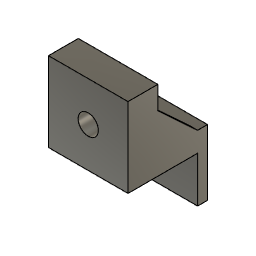
rocker_mount (Autodesk Fusion 360 design; units mm, degrees)
Autodesk Fusion 360 part; units mm, degrees
note: some values were not read from the file. Chosen so that the rebuilt part matches the saved one: a direction.
sketch "Sketch1" plane through (0, 0, 0) normal (1, 0, 0) x (0, 1, 0)
  line L0 (0, 0) -> (35, 0)
  line L1 (35, 0) -> (35, -23)
  line L2 (35, -23) -> (40, -23)
  line L3 (0, 0) -> (0, 10)
  line L4 (15, 30.2) -> (15, 10)
  line L5 (15, 10) -> (40, 10)
  line L6 (40, 10) -> (40, -23)
  line L7 (0, 10) -> (0, 30)
  line L8 (0, 30) -> (0, 40)
  line L9 (0, 40) -> (15, 40)
  line L10 (15, 40) -> (15, 30.2)
  line L11 (15, 10) -> (15, 28.5) construction
  line L12 (15, 28.5) -> (35, 10)
  dimension "d1" = 35
  dimension "d2" = 23
  dimension "d3" = 5
  dimension "d4" = 10
  dimension "d8" = 20.2
  dimension "d9" = 20
  dimension "d10" = 10
  dimension "d19" = 18.5
  constraint coincident L0.start L3.start
  constraint horizontal L0
  constraint perpendicular L0 L1
  constraint perpendicular L1 L2
  constraint perpendicular L0 L3
  constraint perpendicular L0 L4
  constraint perpendicular L4 L5
  constraint perpendicular L2 L6
  constraint parallel L3 L7
  constraint parallel L7 L8
  constraint perpendicular L4 L9
  constraint perpendicular L9 L10
  constraint coincident L4 L11.end
  constraint coincident L5 L12.end
  measures "d1" distance of L0.start L0.end
  measures "d2" distance of L0.end L1.end
  measures "d3" distance of L1.end L2.end
  measures "d4" distance of L0.start L3.end
  measures "d8" distance of L4.start L4.end
  measures "d9" distance of L3.end L7.end
  measures "d10" distance of L7.end L8.end
  measures "d19" distance of L4.end L11.end
extrude "Extrude1" add sketch "Sketch1" along normal blind 40 contours L0 L1 L2 L3 L4 L5 L6 L7 L8 L9 L10
sketch "Sketch2" plane through (0, 0, 0) normal (0, -1, 0) x (1, 0, 0)
  line L0 (0, 40) -> (0, 0)
  line L1 (0, 0) -> (40, 0)
  line L2 (40, 0) -> (40, 40)
  line L3 (40, 40) -> (0, 40)
  line L4 (29.815, 20) -> (24.9075, 28.5)
  line L5 (24.9075, 28.5) -> (15.0925, 28.5)
  line L6 (15.0925, 28.5) -> (10.185, 20)
  line L7 (10.185, 20) -> (15.0925, 11.5)
  line L8 (15.0925, 11.5) -> (24.9075, 11.5)
  line L9 (24.9075, 11.5) -> (29.815, 20)
  line L10 (0, 20) -> (40, 20) construction
  line L11 (20, 40) -> (20, 0) construction
  circle A0 centre (20, 20) radius 5.1
  line L12 (0, 0) -> (0, -11.5) construction
  line L13 (0, -11.5) -> (10, -11.5) construction
  line L14 (10, -11.5) -> (20, -11.5) construction
  circle A1 centre (20, -11.5) radius 2.1
  point P0 (20, 20)
  point P1 (20, 20)
  dimension "d13" = 8.5
  dimension "d14" = 10.2
  dimension "d25" = 11.5
  dimension "d26" = 10
  dimension "d27" = 4.2
  constraint parallel L3 L5
  constraint midpoint L0 L10.start
  constraint midpoint L2 L10.end
  constraint midpoint L3 L11.start
  constraint midpoint L1 L11.end
  constraint midpoint L10 P1
  constraint coincident P1 P0
  constraint coincident L0.end L1.start
  constraint perpendicular L1 L12
  constraint perpendicular L12 L13
  constraint perpendicular L12 L14
  constraint coincident L14.end A1.centre
  measures "d13" distance of P1 L9
  measures "d14" diameter of A0
  measures "d25" distance of L0.end L12.end
  measures "d26" distance of L12.end L13.end
  measures "d27" diameter of A1
extrude "Extrude2" cut sketch "Sketch2" against normal through all contours A0 | A1
extrude "Extrude3" cut sketch "Sketch2" along normal blind 7.5 from surface at -15 contours L4 L5 L6 L7 L8 L9
extrude "Extrude4" add sketch "Sketch1" along normal blind 4 contours L4 L5 L12
extrude "Extrude5" add sketch "Sketch1" against normal blind 4 from surface at 40 contours L4 L5 L12
sketch "Sketch3" plane through (0, 0, 10) normal (0, 0, 1) x (-1, 0, 0)
  line L0 (-36, -35) -> (-40, -35)
  line L1 (-40, -35) -> (-40, -40)
  line L2 (-40, -40) -> (0, -40)
  line L3 (0, -40) -> (0, -35)
  line L4 (0, -35) -> (-4, -35)
  line L5 (-4, -35) -> (-4, -15)
  line L6 (-4, -15) -> (-36, -15)
  line L7 (-36, -15) -> (-36, -35)
  line L8 (0, -40) -> (-10, -40) construction
  line L9 (-10, -40) -> (-10, -27.5) construction
  circle A0 centre (-10, -27.5) radius 1.6
  line L10 (-10, -27.5) -> (-30, -27.5) construction
  circle A1 centre (-30, -27.5) radius 1.6
  dimension "d28" = 10
  dimension "d29" = 12.5
  dimension "d30" = 3.2
  dimension "d31" = 20
  dimension "d32" = 3.2
  constraint coincident L2.end L3.start
  constraint coincident L2 L8.end
  constraint perpendicular L6 L9
  constraint coincident L9.end A0.centre
  constraint perpendicular L7 L10
  constraint coincident L10.end A1.centre
  measures "d28" distance of L2.end L8.end
  measures "d29" distance of L8.end L9.end
  measures "d30" diameter of A0
  measures "d31" distance of L9.end L10.end
  measures "d32" diameter of A1
extrude "Extrude6" cut sketch "Sketch3" against normal through all contours A0 | A1
equation "d8 = 30.200 mm - 10 mm"
equation "d13 = ( 17 / 2 ) * 1 mm"
equation "d19 = 28.50 mm - 10 mm"
equation "d25 = ( 23 / 2 ) * 1 mm"
equation "d29 = ( 25 / 2 ) * 1 mm"
